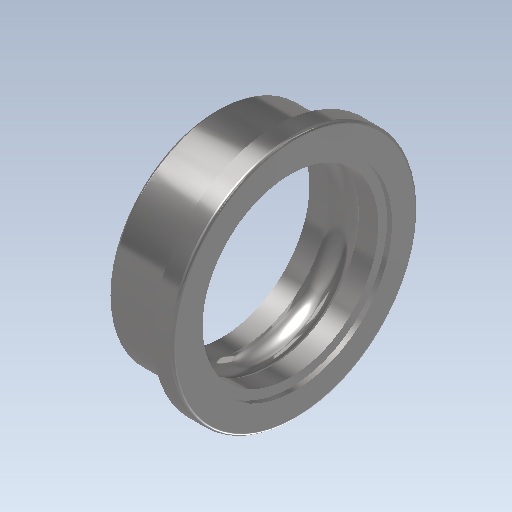
# Autodesk Inventor part: F694ZZ Outer Ring
Saved by Autodesk Inventor 2020 (Build 240168000, 168)
## iProperties
Created: 2018-10-12
Part Number: F694ZZ Outer Ring
Material: ステンレス鋼 440C
Catalog Web Link: www.cadenas.de
Description: shielded_type_zz_zzs_OR-
Vendor: NSK_RB
Document SubType Name: Modeling
Designer: psadmin
Manufacturer: NSK_RB
Mass: 1.07959 g
Surface Area: 3.78987 cm^2
Volume: 0.139303 cm^3
Density: 7.75 g/cm^3
Appearance: 半つや出し
Category: PARTsolutions
Company: NSK_RB
PSOL_IDENT_0: {$CADENAS_DATA\23d-libs\nsk_rb\roller_bearings\deep_groove_bb\exstra_small_miniatur_bb\metric_design
PSOL_IDENT_1: _with_flange\shielded_type_zz_zzs_or1.prj},192 {VTYP=3D},{NB=F694ZZ Outer Ring},{LINA=F694ZZ Outer R
PSOL_IDENT_2: ing},{NN=shielded_type_zz_zzs_OR},{DATE=18.07.2018 08:51:02},{GEOMDATE=04.01.2008 00:00:00},{VERSION=
PSOL_IDENT_3: },{LINEID=250},{WBVAR=},{WBNUMERIC=}  {NB=F694ZZ Outer Ring},{LINA=F694ZZ Outer Ring},{KT=DUMMY},{ID
PSOL_IDENT_4: NR=},{STAN=},{ORDER=F694ZZ},{SD=4.0},{X=4.0},{D=11},{DD=11},{DD1=0.0},{D2=12.5},{DD2=12.5},{B=0.0},{
PSOL_IDENT_5: B1=4.0},{CC1=0.0},{C2=1.0},{CC2=1.0},{R=0.00},{R1=0.15},{DI1=6.15},{DI2=5.60},{SDE1=8.95},{SDE2=9.85
PSOL_IDENT_6: },{CR1=960},{COR1=345},{CR2=98},{COR2=35.0},{LG=48000},{LO=56000},{DA=0.0},{DB=5.6},{RA=0.00},{RB=0.
PSOL_IDENT_7: 15},{MASS=1.96},{SC=1}
NN: shielded_type_zz_zzs_OR
NB: F694ZZ Outer Ring
NBSYN: $ORDER. Outer Ring
LINA: F694ZZ Outer Ring
ORDER: F694ZZ
SD: 4
X: 4
D: 11
DD: 11
DD1: 0
D2: 12.5
DD2: 12.5
B: 0
B1: 4
CC1: 0
C2: 1
CC2: 1
R: 0
R1: 0.15
DI1: 6.15
DI2: 5.6
SDE1: 8.95
SDE2: 9.85
CR1: 960
COR1: 345
CR2: 98
COR2: 35
LG: 48000
LO: 56000
DA: 0
DB: 5.6
RA: 0
RB: 0.15
MASS: 1.96
SC: 1
SUPPLIER: NSK_RB
ARTICLENO: F694ZZ Outer Ring
BOMINFO: F694ZZ Outer Ring
CREATOR: CADENAS GmbH
Title: F694ZZ Outer Ring
Author: Cadenas PARTsolutions
Autodesk Inventor part; units mm, degrees
sketch "Sketch_1" plane through (0, 0, 0) normal (0, 0, 1) x (1, 0, 0)
  line L0 (4, 0) -> (0, 0)
  line L1 (0, 4.925) -> (0.25, 4.925)
  line L2 (0.25, 4.925) -> (0.25, 4.475)
  line L3 (0.25, 4.475) -> (1.2405, 4.475)
  arc A0 (2.7595, 4.475) -> (1.2405, 4.475) centre (2, 3.75) ccw
  line L4 (2.7595, 4.475) -> (3.75, 4.475)
  line L5 (3.75, 4.475) -> (3.75, 4.925)
  line L6 (3.75, 4.925) -> (4, 4.925)
  line L7 (4, 4.925) -> (4, 6.1)
  arc A1 (4, 6.1) -> (3.85, 6.25) centre (3.85, 6.1) ccw
  line L8 (3.85, 6.25) -> (3, 6.25)
  line L9 (3, 6.25) -> (3, 5.5)
  line L10 (3, 5.5) -> (0.15, 5.5)
  arc A2 (0.15, 5.5) -> (0, 5.35) centre (0.15, 5.35) ccw
  line L11 (0, 5.35) -> (0, 4.925)
  constraints: 24 end point, 6 point on circle, 3 centre point
revolve "Revolution1" add sketch "Sketch_1" angle 360 about axis through (4, 0, 0) along (1, 0, 0)
ref_plane "ip_st_1_XY" through (0, 0, 0) normal (1, 0, 0) x (0, 0, -1)
ref_plane "ip_st_1_YZ" through (0, 0, 0) normal (0, 0, -1) x (0, 1, 0)
ref_plane "ip_st_1_ZX" through (0, 0, 0) normal (0, 1, 0) x (1, 0, 0)
ref_plane "ip_st_2_XY" through (3.75, 0, 0) normal (-1, 0, 0) x (0, 0, -1)
ref_plane "ip_st_2_YZ" through (3.75, 0, 0) normal (0, 0, -1) x (0, -1, 0)
ref_plane "ip_st_2_ZX" through (3.75, 0, 0) normal (0, -1, 0) x (-1, 0, 0)
body "Solid1"
